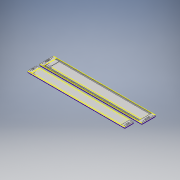
# Autodesk Inventor part: Pedestal Fixture Base
Saved by Autodesk Inventor 2018 (Build 220112000, 112)
## iProperties
Created: 2017-07-11
Part Number: Pedestal Fixture Base
Material: Generic
Document SubType Name: Modeling
Designer: Samuel Clay
Density: 1 g/cm^3
Appearance: Default
Author: Samuel Clay
Autodesk Inventor part; units mm, degrees
ref_plane "YZ Plane" through (0, 0, 0) normal (1, 0, 0) x (0, 1, 0)
ref_plane "XY Plane" through (0, 0, 0) normal (0, 0, 1) x (1, 0, 0)
sketch "Base Sketch" plane through (0, 0, 0) normal (0, 1, 0) x (-1, 0, 0)
  line L0 (0, 0) -> (-50.8, 0)
  line L1 (-1524, 0) -> (-1524, -203.2)
  line L2 (-1524, -203.2) -> (-1473.2, -203.2)
  line L3 (0, -203.2) -> (0, 0)
  line L4 (-50.8, -203.2) -> (-50.8, 0)
  line L5 (-1473.2, -203.2) -> (-1473.2, 0)
  line L6 (-50.8, 0) -> (-1473.2, 0)
  line L7 (-1473.2, 0) -> (-1524, 0)
  line L8 (-50.8, -203.2) -> (0, -203.2)
  line L9 (-1473.2, -203.2) -> (-50.8, -203.2)
  line L10 (0, 50.8) -> (-50.8, 50.8)
  line L11 (-1447.8, 50.8) -> (-1447.8, 177.8)
  line L12 (-1447.8, 177.8) -> (-1397, 177.8)
  line L13 (0, 177.8) -> (0, 50.8)
  line L14 (-50.8, 50.8) -> (-50.8, 177.8)
  line L15 (-1397, 50.8) -> (-1397, 177.8)
  line L16 (-50.8, 50.8) -> (-1397, 50.8)
  line L17 (-1397, 50.8) -> (-1447.8, 50.8)
  line L18 (-50.8, 177.8) -> (0, 177.8)
  line L19 (-1397, 177.8) -> (-50.8, 177.8)
  line L20 (-82.55, 69.85) -> (-1365.25, 69.85) construction
  line L21 (-1365.25, 69.85) -> (-1365.25, 158.75) construction
  line L22 (-1365.25, 158.75) -> (-82.55, 158.75) construction
  line L23 (-82.55, 158.75) -> (-82.55, 69.85) construction
  line L24 (-1384.3, 50.8) -> (-1384.3, 177.8) construction
  line L25 (-63.5, 50.8) -> (-63.5, 177.8) construction
  line L26 (-63.5, 0) -> (-63.5, -203.2) construction
  line L27 (-1460.5, 0) -> (-1460.5, -203.2) construction
  dimension "d0" = 1524
  dimension "d1" = 203.2
  dimension "d2" = 50.8
  dimension "d3" = 50.8
  dimension "d67" = 1447.8
  dimension "d68" = 127
  dimension "d69" = 50.8
  dimension "d70" = 50.8
  dimension "d71" = 50.8
  dimension "d99" = 12.7
  dimension "d100" = 12.7
  dimension "d101" = 19.05
  dimension "d102" = 19.05
  dimension "d103" = 19.05
  dimension "d104" = 19.05
  dimension "d105" = 12.7
  dimension "d106" = 12.7
  constraints: 56 end point, 22 parallel, 22 perpendicular, 10 point on line, 7 horizontal, 1 collinear, 1 vertical
  measures "d0" distance of L3.start L1.end
  measures "d1" distance of L1.end L1.start
  measures "d2" distance between parallel lines of L4 L3
  measures "d3" distance between parallel lines of L1 L5
  measures "d67" distance of L11.end L13.start
  measures "d68" distance of L11.start L11.end
  measures "d69" distance between parallel lines of L10 L6
  measures "d70" distance between parallel lines of L13 L14
  measures "d71" distance between parallel lines of L15 L11
  measures "d99" distance between parallel lines of L25 L14
  measures "d100" distance between parallel lines of L24 L15
  measures "d101" distance between parallel lines of L24 L21
  measures "d102" distance between parallel lines of L25 L23
  measures "d103" distance between parallel lines of L16 L20
  measures "d104" distance between parallel lines of L19 L22
  measures "d105" distance between parallel lines of L5 L27
  measures "d106" distance between parallel lines of L4 L26
extrude "Lower Level" add sketch "Base Sketch" along normal blind 18.796 contours L3 L8 L4 L0 | L5 L2 L1 L7 | L10 L14 L18 L13 | L17 L11 L12 L15
extrude "Base" add sketch "Base Sketch" along normal blind 19.05 contours L4 L9 L5 L6 | L16 L15 L19 L14
sketch "Handles Sketch" plane through (0, 0, 0) normal (0, 1, 0) x (-1, 0, 0)
  line L0 (-19.05, -139.7) -> (-19.05, -63.5) construction
  line L1 (-9.525, -130.175) -> (-9.525, -73.025)
  line L2 (-28.575, -73.025) -> (-28.575, -130.175)
  arc A0 (-28.575, -130.175) -> (-9.525, -130.175) centre (-19.05, -130.175) ccw
  arc A1 (-9.525, -73.025) -> (-28.575, -73.025) centre (-19.05, -73.025) ccw
  line L3 (-1524, -203.2) -> (0, -203.2) projected
  line L4 (0, 0) -> (-1524, 0) projected
  line L5 (0, -203.2) -> (0, 0) projected
  line L6 (-1524, 0) -> (-1524, -203.2) projected
  line L7 (-1504.95, -139.7) -> (-1504.95, -63.5) construction
  line L8 (-1495.425, -130.175) -> (-1495.425, -73.025)
  line L9 (-1514.475, -73.025) -> (-1514.475, -130.175)
  arc A2 (-1514.475, -130.175) -> (-1495.425, -130.175) centre (-1504.95, -130.175) ccw
  arc A3 (-1495.425, -73.025) -> (-1514.475, -73.025) centre (-1504.95, -73.025) ccw
  line L10 (0, 177.8) -> (-1447.8, 177.8) projected
  line L11 (-1447.8, 50.8) -> (0, 50.8) projected
  line L12 (0, 50.8) -> (0, 177.8) projected
  line L13 (-1447.8, 177.8) -> (-1447.8, 50.8) projected
  line L14 (-19.05, 139.7) -> (-19.05, 88.9) construction
  line L15 (-28.575, 130.175) -> (-28.575, 98.425)
  line L16 (-9.525, 98.425) -> (-9.525, 130.175)
  arc A4 (-9.525, 130.175) -> (-28.575, 130.175) centre (-19.05, 130.175) ccw
  arc A5 (-28.575, 98.425) -> (-9.525, 98.425) centre (-19.05, 98.425) ccw
  line L17 (-1428.75, 139.7) -> (-1428.75, 88.9) construction
  line L18 (-1438.275, 130.175) -> (-1438.275, 98.425)
  line L19 (-1419.225, 98.425) -> (-1419.225, 130.175)
  arc A6 (-1419.225, 130.175) -> (-1438.275, 130.175) centre (-1428.75, 130.175) ccw
  arc A7 (-1438.275, 98.425) -> (-1419.225, 98.425) centre (-1428.75, 98.425) ccw
  point P0 (-19.05, -177.8)
  point P1 (-19.05, -158.75)
  point P2 (-19.05, -44.45)
  point P3 (-19.05, -25.4)
  point P4 (-1504.95, -25.4)
  point P5 (-1504.95, -44.45)
  point P6 (-1504.95, -158.75)
  point P7 (-1504.95, -177.8)
  point P8 (-19.05, -101.6)
  point P9 (-1504.95, -101.6)
  point P10 (-19.05, 63.5)
  point P11 (-19.05, 76.2)
  point P12 (-19.05, 152.4)
  point P13 (-19.05, 165.1)
  point P14 (-1428.75, 165.1)
  point P15 (-1428.75, 152.4)
  point P16 (-1428.75, 76.2)
  point P17 (-1428.75, 63.5)
  point P18 (-19.05, 114.3)
  point P19 (-1428.75, 114.3)
  dimension "d5" = 19.05
  dimension "d6" = 25.4
  dimension "d7" = 19.05
  dimension "d8" = 19.05
  dimension "d9" = 19.05
  dimension "d10" = 19.05
  dimension "d11" = 19.05
  dimension "d12" = 25.4
  dimension "d13" = 19.05
  dimension "d14" = 76.2
  dimension "d15" = 19.05
  dimension "d16" = 19.05
  dimension "d17" = 19.05
  dimension "d18" = 25.4
  dimension "d19" = 19.05
  dimension "d21" = 19.05
  dimension "d22" = 19.05
  dimension "d25" = 19.05
  dimension "d26" = 19.05
  dimension "d27" = 19.05
  dimension "d28" = 25.4
  dimension "d29" = 19.05
  dimension "d30" = 19.05
  dimension "d31" = 19.05
  dimension "d32" = 76.2
  dimension "d72" = 12.7
  dimension "d73" = 12.7
  dimension "d74" = 12.7
  dimension "d75" = 12.7
  dimension "d76" = 19.05
  dimension "d77" = 19.05
  dimension "d78" = 12.7
  dimension "d79" = 12.7
  dimension "d80" = 12.7
  dimension "d81" = 12.7
  dimension "d83" = 19.05
  dimension "d84" = 12.7
  dimension "d85" = 12.7
  dimension "d86" = 19.05
  dimension "d87" = 12.7
  dimension "d88" = 12.7
  constraints: 32 end point, 24 point on circle, 16 tangent, 9 vertical alignment, 8 centre point, 8 point on line, 4 midpoint, 4 parallel, 3 vertical
  measures "d5" diameter of A1
  measures "d6" distance from line of point (-19.05, -177.8) L3
  measures "d7" distance from line of L5 point (-19.05, -177.8)
  measures "d8" distance of point (-19.05, -177.8) point (-19.05, -158.75)
  measures "d9" distance from line of L5 point (-19.05, -158.75)
  measures "d10" distance from line of L5 point (-19.05, -44.45)
  measures "d11" distance from line of L5 point (-19.05, -25.4)
  measures "d12" distance from line of L4 point (-19.05, -25.4)
  measures "d13" distance of point (-19.05, -25.4) point (-19.05, -44.45)
  measures "d14" distance of L0.start L0.end
  measures "d15" distance of point (-19.05, -158.75) L0.start
  measures "d16" distance of point (-19.05, -44.45) L0.end
  measures "d17" distance from line of L5 point (-19.05, -101.6)
  measures "d18" distance from line of point (-1504.95, -177.8) L3
  measures "d19" distance of point (-1504.95, -158.75) point (-1504.95, -177.8)
  measures "d21" distance from line of L6 point (-1504.95, -177.8)
  measures "d22" distance from line of L6 point (-1504.95, -158.75)
  measures "d25" distance of point (-1504.95, -25.4) point (-1504.95, -44.45)
  measures "d26" distance from line of L6 point (-1504.95, -44.45)
  measures "d27" distance from line of L6 point (-1504.95, -25.4)
  measures "d28" distance from line of L4 point (-1504.95, -25.4)
  measures "d29" diameter of A3
  measures "d30" distance of point (-1504.95, -158.75) L7.start
  measures "d31" distance of L7.end point (-1504.95, -44.45)
  measures "d32" distance of L7.end L7.start
  measures "d72" distance from line of L10 point (-19.05, 165.1)
  measures "d73" distance of point (-19.05, 152.4) point (-19.05, 165.1)
  measures "d74" distance from line of L11 point (-19.05, 63.5)
  measures "d75" distance of point (-19.05, 63.5) point (-19.05, 76.2)
  measures "d76" distance from line of L12 point (-19.05, 165.1)
  measures "d77" distance from line of L13 point (-1428.75, 165.1)
  measures "d78" distance from line of L10 point (-1428.75, 165.1)
  measures "d79" distance of point (-1428.75, 165.1) point (-1428.75, 152.4)
  measures "d80" distance of point (-1428.75, 63.5) point (-1428.75, 76.2)
  measures "d81" distance from line of L11 point (-1428.75, 63.5)
  measures "d83" diameter of A5
  measures "d84" distance of L14.start point (-19.05, 152.4)
  measures "d85" distance of point (-19.05, 76.2) L14.end
  measures "d86" diameter of A7
  measures "d87" distance of L17.start point (-1428.75, 152.4)
  measures "d88" distance of point (-1428.75, 76.2) L17.end
extrude "Extrusion3" cut sketch "Handles Sketch" along normal through all contours A0 L2 A1 L1 | A2 L9 A3 L8 | A4 L16 A5 L15 | A6 L19 A7 L18
hole "Hole1" at (19.05, 0, 165.1) at (19.05, 0, 152.4) at (19.05, 0, 76.2) at (19.05, 0, 63.5) at (19.05, 0, -25.4) at (19.05, 0, -44.45) at (19.05, 0, -158.75) at (19.05, 0, -177.8) at (1428.75, 0, 165.1) at (1428.75, 0, 152.4) at (1428.75, 0, 76.2) at (1428.75, 0, 63.5) at (1504.95, 0, -25.4) at (1504.95, 0, -44.45) at (1504.95, 0, -158.75) at (1504.95, 0, -177.8) direction (0, 1, 0) diameter 6.35 end through all
ref_plane "Work Plane1" through (50.8, 19.05, 0) normal (0, 1, 0) x (-1, 0, 0)
sketch "Pocket Level Sketch" plane through (0, 19.05, 0) normal (0, 1, 0) x (1, 0, 0)
  line L0 (1473.2, 203.2) -> (1473.2, 0) projected
  line L1 (50.8, 6.35) -> (1473.2, 6.35)
  line L2 (1473.2, 6.35) -> (1473.2, 25.908)
  line L3 (1473.2, 25.908) -> (50.8, 25.908)
  line L4 (50.8, 25.908) -> (50.8, 6.35)
  line L5 (50.8, 203.2) -> (50.8, 0) projected
  line L6 (50.8, 196.85) -> (1473.2, 196.85)
  line L7 (1473.2, 196.85) -> (1473.2, 177.292)
  line L8 (1473.2, 177.292) -> (50.8, 177.292)
  line L9 (50.8, 177.292) -> (50.8, 196.85)
  line L10 (1473.2, 203.2) -> (50.8, 203.2) projected
  line L11 (50.8, 0) -> (1473.2, 0) projected
  line L12 (114.3, 44.958) -> (1473.2, 44.958)
  line L13 (1473.2, 44.958) -> (1473.2, 177.292)
  line L14 (1473.2, 177.292) -> (114.3, 177.292)
  line L15 (114.3, 177.292) -> (114.3, 44.958)
  circle A0 centre (118.745, 49.403) radius 12.7
  point P0 (0, 0)
  dimension "d39" = 19.558
  dimension "d40" = 6.35
  dimension "d41" = 19.558
  dimension "d42" = 6.35
  dimension "d44" = 63.5
  dimension "d45" = 19.05
  dimension "d50" = 25.4
  dimension "d51" = 4.445
  dimension "d52" = 4.445
  constraints: 24 end point, 6 parallel, 3 collinear, 3 horizontal, 3 perpendicular, 3 point on line, 1 centre point
  measures "d39" distance of L2.end L1.end
  measures "d40" distance between parallel lines of L6 L10
  measures "d41" distance between parallel lines of L6 L8
  measures "d42" distance between parallel lines of L11 L1
  measures "d44" distance between parallel lines of L5 L15
  measures "d45" distance between parallel lines of L3 L12
  measures "d50" diameter of A0
  measures "d51" distance from line of L12 A0.centre
  measures "d52" distance from line of L15 A0.centre
extrude "Bed Cut" cut sketch "Pocket Level Sketch" against normal blind 3.175 contours L0 L12 A0 L15 L8 | A0 L15 L12 | L12 L15 A0
extrude "Tracks Cut" cut sketch "Pocket Level Sketch" against normal blind 10.16 contours L0 L8 L5 L6 | L0 L1 L4 L3
sketch "Origin Sketch" plane through (50.8, 19.05, 0) normal (0, 1, 0) x (-1, 0, 0)
  line L0 (-12.7, 50.8) -> (-12.7, 177.8) construction
  line L1 (-31.75, 158.75) -> (-31.75, 69.85) construction
  line L2 (-1314.45, 158.75) -> (-31.75, 158.75) construction
  line L3 (-31.75, 69.85) -> (-1314.45, 69.85) construction
  line L4 (-1314.45, 69.85) -> (-1314.45, 158.75) construction
  line L5 (-1333.5, 50.8) -> (-1333.5, 177.8) construction
  line L6 (-12.7, 0) -> (-12.7, -203.2) construction
  line L7 (-1409.7, 0) -> (-1409.7, -203.2) construction
  line L8 (0, -203.2) -> (0, 0) projected
  line L9 (50.8, 0) -> (-1473.2, 0) projected
  line L10 (-1473.2, -203.2) -> (50.8, -203.2) projected
  line L11 (0, 50.8) -> (-1346.2, 50.8) projected
  line L12 (0, 50.8) -> (0, 177.8) projected
  line L13 (50.8, 177.8) -> (-1397, 177.8) projected
  line L14 (-1422.4, -44.958) -> (-79.8417, -44.958) projected
  point P0 (-12.7, -44.958)
  point P1 (-19.05, 171.45)
  dimension "d107" = 0
  dimension "d109" = 6.35
  dimension "d110" = 6.35
  constraints: 1 point on line
  measures "d107" distance from line of L6 point (-12.7, -44.958)
  measures "d109" distance from line of L0 point (-19.05, 171.45)
  measures "d110" distance from line of L13 point (-19.05, 171.45)
sketch "Registration Sketch" plane through (50.8, 19.05, 0) normal (0, 1, 0) x (-1, 0, 0)
  circle A0 centre (-12.7, -44.958) radius 3.175
  circle A1 centre (-19.05, 171.45) radius 3.175
  point P0 (50.8, 0)
  dimension "d96" = 6.35
  dimension "d111" = 6.35
  constraints: 2 centre point, 2 coincident
  measures "d96" diameter of A0
  measures "d111" diameter of A1
extrude "Registration Hole" cut sketch "Registration Sketch" against normal blind 1.27
equation "\"d70\" = d2"
equation "\"d71\" = d3"
equation "\"d100\" = d99"
equation "\"d102\" = d101"
equation "\"d103\" = d102"
equation "\"d104\" = d102"
equation "\"d105\" = d100"
equation "\"d106\" = d99"
equation "\"d7\" = d17"
equation "\"d10\" = d7"
equation "\"d11\" = d10"
equation "\"d12\" = d6"
equation "\"d13\" = d8"
equation "\"d15\" = d8"
equation "\"d16\" = d13"
equation "\"d17\" = d9"
equation "\"d18\" = d6"
equation "\"d19\" = d8"
equation "\"d21\" = d9"
equation "\"d22\" = d21"
equation "\"d25\" = d13"
equation "\"d26\" = d22"
equation "\"d27\" = d21"
equation "\"d28\" = d12"
equation "\"d30\" = d19"
equation "\"d31\" = d30"
equation "\"d32\" = d14"
equation "\"d74\" = d72"
equation "\"d75\" = d73"
equation "\"d77\" = d76"
equation "\"d78\" = d72"
equation "\"d79\" = d73"
equation "\"d80\" = d75"
equation "\"d81\" = d74"
equation "\"d85\" = d84"
equation "\"d87\" = d84"
equation "\"d88\" = d85"
equation "\"d40\" = d42"
equation "\"d41\" = d39"
equation "\"d52\" = d51"
body "Solid1"
